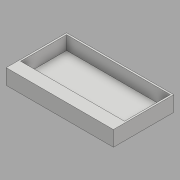
# Autodesk Inventor part: Battery Case Bottom
Saved by Autodesk Inventor 2017 (Build 210142000, 142)
## iProperties
Created: 2017-05-07
Part Number: Battery Case Bottom
Material: Generic
Document SubType Name: Modeling
Designer: zallen
Density: 1 g/cm^3
Appearance: Default
Author: zallen
Autodesk Inventor part; units mm, degrees
ref_plane "YZ Plane" through (0, 0, 0) normal (1, 0, 0) x (0, 1, 0)
ref_plane "XZ Plane" through (0, 0, 0) normal (0, 1, 0) x (-1, 0, 0)
ref_plane "XY Plane" through (0, 0, 0) normal (0, 0, 1) x (1, 0, 0)
sketch "Sketch1" plane through (0, 0, 0) normal (0, 0, 1) x (1, 0, 0)
  line L0 (0, 0) -> (126, 0)
  line L1 (126, 0) -> (126, 71)
  line L2 (126, 71) -> (0, 71)
  line L3 (0, 71) -> (0, 0)
  dimension "d0" = 126
  dimension "d1" = 71
  constraints: 8 end point, 2 parallel, 1 horizontal, 1 perpendicular
  measures "d0" distance of L2.end L1.end
  measures "d1" distance of L1.end L0.end
extrude "Extrusion1" add sketch "Sketch1" along normal blind 2
sketch "Sketch2" plane through (0, 0, 2) normal (0, 0, 1) x (1, 0, 0)
  line L0 (126, 0) -> (126, 71) projected
  line L1 (0, 0) -> (126, 0)
  line L2 (126, 0) -> (126, 15)
  line L3 (126, 15) -> (0, 15)
  line L4 (0, 15) -> (0, 0)
  line L5 (0, 71) -> (2, 71)
  line L6 (2, 71) -> (2, 15)
  line L7 (2, 15) -> (0, 15)
  line L8 (0, 15) -> (0, 71)
  line L9 (126, 71) -> (124, 71)
  line L10 (124, 71) -> (124, 15)
  line L11 (124, 15) -> (126, 15)
  line L12 (126, 15) -> (126, 71)
  line L13 (2, 71) -> (124, 71)
  line L14 (124, 71) -> (124, 69)
  line L15 (124, 69) -> (2, 69)
  line L16 (2, 69) -> (2, 71)
  dimension "d4" = 15
  dimension "d7" = 2
  dimension "d8" = 2
  dimension "d9" = 2
  dimension "d11" = 122
  dimension "d14" = 54
  constraints: 32 end point, 8 parallel, 4 horizontal, 4 perpendicular, 4 point on line
  measures "d4" distance of L2.end L1.end
  measures "d7" distance of L6.end L7.end
  measures "d8" distance of L11.end L10.end
  measures "d9" distance of L13.end L14.end
  measures "d11" distance between parallel lines of L10 L6
  measures "d14" distance between parallel lines of L3 L15
extrude "Extrusion3" add sketch "Sketch2" along normal blind 16 contours L1 L4 L3 L0 | L3 L10 L9 L0 | L8 L5 L6 L3 | L10 L15 L6 L13
body "Solid1"
